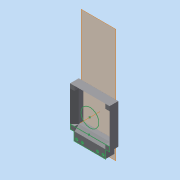
# Autodesk Inventor part: 09_Opentrons_Autofocus_LED_Module
Saved by Autodesk Inventor 2019.4 (Build 234330000, 330)
## iProperties
Created: 2020-11-27
Part Number: 09_Opentrons_Autofocus_LED_Module
Material: Generic
Document SubType Name: Modeling
Designer: diederichbenedict
Density: 1 g/cm^3
Appearance: Default
Author: diederichbenedict
Autodesk Inventor part; units mm, degrees
ref_plane "YZ Plane" through (0, 0, 0) normal (1, 0, 0) x (0, 1, 0)
ref_plane "XZ Plane" through (0, 0, 0) normal (0, 1, 0) x (-1, 0, 0)
ref_plane "XY Plane" through (0, 0, 0) normal (0, 0, 1) x (1, 0, 0)
ref_plane "Work Plane1" through (0, 0, 0) normal (0, 0, 1) x (1, 0, 0)
sketch "Sketch1" plane through (0, 0, 0) normal (0, 0, 1) x (1, 0, 0)
  circle A0 centre (8.8475, 49.7489) radius 1.45 construction
  circle A1 centre (9.593, -3.6603) radius 1.45 construction
  circle A2 centre (-7.7223, -3.6603) radius 1.45 construction
  circle A3 centre (-14.1116, -11.6603) radius 1.45 construction
  circle A4 centre (-7.7223, -11.6603) radius 1.45 construction
  circle A5 centre (9.593, -11.6603) radius 1.45 construction
  circle A6 centre (15.9823, -11.6603) radius 1.45 construction
  circle A7 centre (-6.9768, 49.7489) radius 1.45 construction
  line L0 (-13.863, 30.0397) -> (-13.8585, 17.3397) construction
  line L1 (-6.6783, 30.0397) -> (-13.863, 30.0397) construction
  arc A8 (15.6915, 17.3397) -> (-6.6783, 30.0397) centre (0.9353, 17.3993) ccw construction
  arc A9 (-6.6783, 4.6397) -> (15.6915, 17.3397) centre (0.9353, 17.2801) ccw construction
  line L2 (-6.6783, 4.6397) -> (-13.863, 4.6397) construction
  line L3 (-13.863, 4.6397) -> (-13.8585, 17.3397) construction
  line L4 (-17.1585, 69.3865) -> (-2.1585, 69.3865) construction
  line L5 (-2.1585, 69.3865) -> (-2.1585, 62.7008) construction
  line L6 (-2.1585, 62.7008) -> (-2.1585, 59.9787) construction
  line L7 (-2.1585, 59.9787) -> (-2.1585, 53.293) construction
  line L8 (-2.1585, 53.293) -> (-17.1585, 53.293) construction
  line L9 (-17.1585, 53.293) -> (-17.1585, -14.6603) construction
  line L10 (-17.1585, -14.6603) -> (18.8415, -14.6603) construction
  line L11 (18.8415, -14.6603) -> (18.8415, 91.3397) construction
  line L12 (-6.8647, 91.3397) -> (18.8415, 91.3397) construction
  line L13 (-6.8647, 103.3397) -> (-6.8647, 91.3397) construction
  line L14 (-17.1585, 103.3397) -> (-6.8647, 103.3397) construction
  line L15 (-17.1585, 69.3865) -> (-17.1585, 103.3397) construction
  line L16 (18.4353, 34.7801) -> (-16.5647, 34.7801)
  line L17 (-16.5647, 34.7801) -> (-16.5647, -0.2199)
  line L18 (-16.5647, -0.2199) -> (18.4353, -0.2199)
  line L19 (18.4353, -0.2199) -> (18.4353, 34.7801)
  line L20 (18.4353, 34.7801) -> (-16.5647, -0.2199) construction
  line L21 (-16.5647, 34.7801) -> (18.4353, -0.2199) construction
  line L22 (23.4353, -5.2199) -> (-21.5647, -5.2199)
  line L23 (-21.5647, -5.2199) -> (-21.5647, 39.7801)
  line L24 (-21.5647, 39.7801) -> (23.4353, 39.7801)
  line L25 (23.4353, 39.7801) -> (23.4353, -5.2199)
  line L26 (23.4353, -5.2199) -> (-21.5647, 39.7801) construction
  line L27 (-21.5647, -5.2199) -> (23.4353, 39.7801) construction
  line L28 (-17.1585, -14.6603) -> (18.8415, -14.6603)
  line L29 (18.8415, -14.6603) -> (18.8415, -5.2199)
  line L30 (18.8415, -5.2199) -> (-17.1585, -5.2199)
  line L31 (-17.1585, -5.2199) -> (-17.1585, -14.6603)
  circle A10 centre (-14.1116, -11.6603) radius 1.45
  circle A11 centre (-7.7223, -11.6603) radius 1.45
  circle A12 centre (9.593, -11.6603) radius 1.45
  circle A13 centre (15.9823, -11.6603) radius 1.45
  point P0 (0, 0)
  dimension "d0" = 35
  dimension "d1" = 35
  dimension "d2" = 45
  dimension "d3" = 45
  constraints: 32 end point, 6 parallel, 4 centre point, 4 coincident, 4 concentric, 4 midpoint, 3 horizontal, 3 perpendicular, 2 point on line
  measures "d0" distance of L18.end L17.end
  measures "d1" distance of L17.end L16.end
  measures "d2" distance of L23.end L24.end
  measures "d3" distance of L22.end L23.end
extrude "Extrusion1" add sketch "Sketch1" along normal blind 10
sketch "Sketch2" plane through (-16.5647, 34.7801, 0) normal (0, -1, 0) x (1, 0, 0)
  line L0 (0, 0) -> (0, 10) projected
  line L1 (35, 0) -> (0, 0) projected
  line L2 (35, 0) -> (35, 10) projected
  line L3 (0, 10) -> (35, 10) projected
  line L4 (0, 0) -> (0, 10) projected
  line L5 (5, 0) -> (-5, 10)
  line L6 (5, 0) -> (19.1421, 0) construction
  line L7 (-5, 10) -> (5, 10)
  line L8 (40, 10) -> (-5, 10) projected
  line L9 (5, 0) -> (5, 10)
  line L10 (-5, 0) -> (-5, 10) projected
  line L11 (12.5, -7.6051) -> (12.5, -58.2325)
  line L12 (40, 10) -> (30, 0)
  line L13 (40, 0) -> (-5, 0) projected
  line L14 (40, 10) -> (54.1421, 10) construction
  line L15 (30, 0) -> (40, 10)
  line L16 (30, 0) -> (30, 10)
  line L17 (30, 0) -> (40, 0) construction
  line L18 (30, 10) -> (40, 10)
  point P0 (16.5647, 0)
  dimension "d6" = 135
  dimension "d7" = 10
  dimension "d9" = 45
  dimension "d10" = 0
  dimension "d11" = 135
  dimension "d12" = 90
  constraints: 22 end point, 3 equal length, 3 horizontal, 2 point on line, 1 collinear, 1 perpendicular, 1 vertical, 4 other
  measures "d6" angle of L6 L5
  measures "d7" distance of L7.end L5.start
  measures "d9" angle of L7 L5
  measures "d10" distance from line of L10 L5.end
  measures "d11" angle of L12 L14
  measures "d12" angle of L17 L16
extrude "Extrusion2" cut sketch "Sketch2" along normal up to surface (35 mm away) contours L5 L7 L0 | L0 L3 L9 L5 | L9 L3 L16 L1 | L16 L3 L2 L12 | L2 L8 L12
sketch "Sketch3" plane through (0, 0, 10) normal (0, 0, 1) x (1, 0, 0)
  line L0 (23.4353, -0.2199) -> (-21.5647, -0.2199) projected
  line L1 (-21.5647, -0.2199) -> (-21.5647, -5.2199) projected
  line L2 (-21.5647, -5.2199) -> (-17.1585, -5.2199) projected
  line L3 (-17.1585, -5.2199) -> (-17.1585, -14.6603) projected
  line L4 (-17.1585, -14.6603) -> (18.8415, -14.6603) projected
  line L5 (18.8415, -14.6603) -> (18.8415, -5.2199) projected
  line L6 (18.8415, -5.2199) -> (23.4353, -5.2199) projected
  line L7 (23.4353, -5.2199) -> (23.4353, -0.2199) projected
  circle A0 centre (15.9823, -11.6603) radius 1.45 projected
  circle A1 centre (9.593, -11.6603) radius 1.45 projected
  circle A2 centre (-7.7223, -11.6603) radius 1.45 projected
  circle A3 centre (-14.1116, -11.6603) radius 1.45 projected
  circle A4 centre (0.9353, 17.3993) radius 10.125 projected
  point P0 (0, 0)
ref_plane "Work Plane2" through (0.9353, 17.3993, 8.4308) normal (0, 0, 1) x (1, 0, 0)
pattern_circular "Circular Pattern1" count 2 over 90 about axis through (0.9353, 17.3993, 10) along (0, 0, 1) of "Extrusion2"
sketch "Sketch4" plane through (0, 0, 10) normal (0, 0, 1) x (1, 0, 0)
  line L0 (-16.4454, -5.1007) -> (-16.4454, -0.2199) projected
  line L1 (-16.4454, -0.2199) -> (-21.5647, -0.2199) projected
  line L2 (-21.5647, -0.2199) -> (-21.5647, -5.2199) projected
  line L3 (-21.5647, -5.2199) -> (-17.1585, -5.2199) projected
  line L4 (-17.1585, -5.2199) -> (-17.1585, -14.6603) projected
  line L5 (-17.1585, -14.6603) -> (18.8415, -14.6603) projected
  line L6 (18.8415, -14.6603) -> (18.8415, -5.2199) projected
  line L7 (18.8415, -5.2199) -> (23.4353, -5.2199) projected
  line L8 (23.4353, -5.2199) -> (23.4353, -0.2199) projected
  line L9 (23.4353, -0.2199) -> (18.5546, -0.2199) projected
  line L10 (18.5546, -0.2199) -> (18.5546, -5.1007) projected
  line L11 (18.5546, -5.1007) -> (-16.4454, -5.1007) projected
  circle A0 centre (15.9823, -11.6603) radius 1.45 projected
  circle A1 centre (9.593, -11.6603) radius 1.45 projected
  circle A2 centre (-7.7223, -11.6603) radius 1.45 projected
  circle A3 centre (-14.1116, -11.6603) radius 1.45 projected
  point P0 (0, 0)
hole "Hole1" at (-14.1116, -11.6603, 10) at (-7.7223, -11.6603, 10) at (9.593, -11.6603, 10) at (15.9823, -11.6603, 10) direction (0, 0, -1) diameter 2.9 end through all counterbore diameter 6 counterbore depth 7
body "Solid1"
